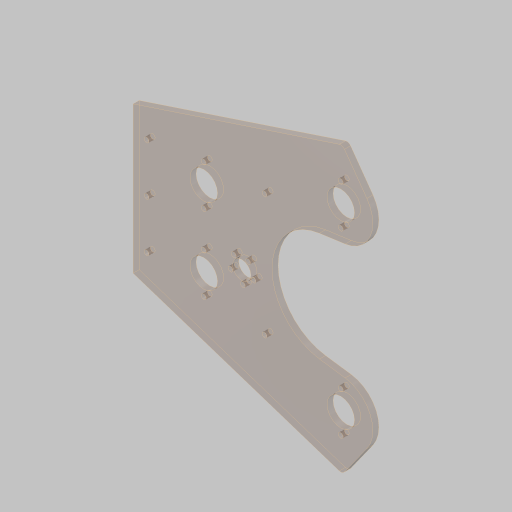
# Autodesk Inventor part: Part1
Saved by Autodesk Inventor 2023.5 (Build 275446000, 446)
## iProperties
Created: 2025-02-23
Part Number: Part1
Material: Polycarbonate, Smoke
Document SubType Name: Modeling
Designer: slick
Density: 1.2 g/cm^3
Appearance: Polycarbonate - Smoked
Author: slick
Autodesk Inventor part; units mm, degrees
ref_plane "YZ Plane" through (0, 0, 0) normal (1, 0, 0) x (0, 1, 0)
ref_plane "XZ Plane" through (0, 0, 0) normal (0, 1, 0) x (-1, 0, 0)
ref_plane "XY Plane" through (0, 0, 0) normal (0, 0, 1) x (1, 0, 0)
sketch "Sketch1" plane through (0, 0, 0) normal (0, 0, 1) x (1, 0, 0)
  circle A0 centre (0, 93.3256) radius 38.1 construction
  circle A1 centre (0, -93.3256) radius 38.1 construction
  line L0 (0, 93.3256) -> (0, -93.3256) construction
  circle A2 centre (-19.05, 0) radius 57.15 construction
  circle A3 centre (0, 93.3256) radius 14.2875
  circle A4 centre (0, -93.3256) radius 14.2875
  circle A5 centre (0, -93.3256) radius 33.3375 construction
  circle A6 centre (0, 93.3256) radius 33.3375 construction
  circle A7 centre (-142.4318, -39.6875) radius 14.3256 construction
  circle A8 centre (0, -93.3256) radius 23.876 construction
  line L1 (-142.4318, -39.6875) -> (0, -93.3256) construction
  circle A9 centre (-142.4318, 39.6875) radius 14.3256 construction
  circle A10 centre (0, 93.3256) radius 23.876 construction
  line L2 (0, 93.3256) -> (-142.4318, 39.6875) construction
  circle A11 centre (-142.4318, 39.6875) radius 39.6875 construction
  circle A12 centre (-142.4318, -39.6875) radius 39.6875 construction
  line L3 (-142.4318, 39.6875) -> (-142.4318, -39.6875) construction
  line L4 (-138.2343, 25.9906) -> (6.9958, 70.4975) construction
  line L5 (-9.8, 115.0976) -> (-148.3118, 52.7507) construction
  line L6 (-138.2343, -25.9906) -> (6.9958, -70.4975) construction
  line L7 (-13.7535, -112.8423) -> (-134.1797, -27.9775) construction
  circle A13 centre (-142.4318, 39.6875) radius 14.2875
  circle A14 centre (-142.4318, -39.6875) radius 14.2875
  circle A15 centre (-102.9059, -16.8672) radius 5.9531 construction
  circle A16 centre (-102.9059, -16.8672) radius 9.525
  circle A17 centre (-102.9059, -16.8672) radius 12.7 construction
  circle A18 centre (-102.9059, -16.8672) radius 12.7 construction
  circle A19 centre (-102.9059, -16.8672) radius 12.7 construction
  circle A20 centre (-102.9059, -16.8672) radius 12.7 construction
  circle A21 centre (-102.9059, -16.8672) radius 12.7 construction
  circle A22 centre (-14.2875, 0) radius 57.15 construction
  circle A23 centre (-102.9059, -16.8672) radius 19.05 construction
  line L8 (-215.9, 76.2) -> (-190.5, 76.2) construction
  line L9 (-190.5, 76.2) -> (-190.5, -76.2) construction
  line L10 (-190.5, -76.2) -> (-215.9, -76.2) construction
  line L11 (-215.9, -76.2) -> (-215.9, 76.2)
  line L12 (-142.4318, -39.6875) -> (-102.9059, -16.8672) construction
  line L13 (-79.1995, 63.5) -> (-79.1995, -63.5) construction
  line L14 (-22.1185, -56.6109) -> (4.5681, -60.3025)
  arc A24 (4.5681, 60.3025) -> (27.142, 112.6828) centre (0, 93.3256) ccw
  arc A25 (-22.1185, 56.6109) -> (-22.1185, -56.6109) centre (-14.2875, 0) ccw
  line L15 (4.5681, 60.3025) -> (-22.1185, 56.6109)
  arc A26 (27.142, -112.6828) -> (4.5681, -60.3025) centre (0, -93.3256) ccw
  arc A27 (3.8774, 145.3034) -> (-1.4945, 147.06) centre (0, 142.5381) ccw
  circle A28 centre (0, 93.3256) radius 44.45 construction
  line L16 (3.8774, 145.3034) -> (27.142, 112.6828)
  line L17 (-1.4945, 147.06) -> (-215.9, 76.2)
  arc A29 (-1.4945, -147.06) -> (3.8774, -145.3034) centre (0, -142.5381) ccw
  line L18 (-215.9, -76.2) -> (-1.4945, -147.06)
  line L19 (27.142, -112.6828) -> (3.8774, -145.3034)
  circle A30 centre (0, -93.3256) radius 44.45 construction
  line L20 (0, 114.3441) -> (0, 72.3071) construction
  line L21 (-142.4318, 60.706) -> (-142.4318, 18.669) construction
  line L22 (-142.4318, -18.669) -> (-142.4318, -60.706) construction
  line L23 (0, -72.3071) -> (0, -114.3441) construction
  line L24 (-201.797, 50.8) -> (-201.797, -50.8) construction
  point P0 (0, 0)
  point P1 (0, 0)
  point P2 (-111.2471, -7.2904)
  point P3 (-114.5915, -21.8408)
  point P4 (-101.7868, -29.5178)
  point P5 (-90.5286, -19.7121)
  point P6 (-96.3754, -5.9749)
  point P7 (-190.5, 0)
  point P8 (-201.797, 0)
  point P9 (-201.797, 0)
  dimension "d15" = 25.4
  dimension "d0" = 76.2
  dimension "d1" = 76.2
  dimension "d2" = 114.3
  dimension "d4" = 186.6511
  dimension "d5" = 28.575
  dimension "d6" = 19.05
  dimension "d7" = 28.6512
  dimension "d8" = 47.752
  dimension "d9" = 79.375
  dimension "d10" = 142.4318
  dimension "d11" = 152.1968
  dimension "d12" = 28.575
  dimension "d13" = 11.9062
  dimension "d14" = 19.05
  dimension "d18" = 360
  dimension "d20" = 4.7625
  dimension "d21" = 38.1
  dimension "d22" = 25.4
  dimension "d23" = 152.4
  dimension "d24" = 215.9
  dimension "d25" = 60
  dimension "d26" = 127
  dimension "d29" = 9.525
  dimension "d30" = 6.35
  dimension "d32" = 42.037
  dimension "d33" = 42.037
  dimension "d34" = 42.037
  dimension "d35" = 42.037
  dimension "d36" = 19.05
  dimension "d44" = 101.6
  constraints: 50 end point, 26 centre point, 24 point on circle, 24 tangent, 16 coincident, 9 equal radius, 8 vertical, 7 midpoint, 3 horizontal alignment, 2 parallel, 2 point on line, 2 vertical alignment, 1 equal length, 1 horizontal, 1 perpendicular, 31 other
  measures "d0" diameter of A0
  measures "d1" diameter of A1
  measures "d2" diameter of A2
  measures "d4" distance of L0.end L0.start
  measures "d5" diameter of A3
  measures "d6" radial gap between concentric circles of A4 A5
  measures "d7" diameter of A7
  measures "d8" diameter of A8
  measures "d9" diameter of A11
  measures "d10" distance from line of L0.start L3
  measures "d11" distance of L2.end L2.start
  measures "d12" diameter of A13
  measures "d13" diameter of A15
  measures "d14" diameter of A16
  measures "d20" distance of A2.centre A22.centre
  measures "d21" diameter of A23
  measures "d22" distance of L9.end L10.end
  measures "d23" distance of L10.end L8.start
  measures "d24" distance from line of A3.centre L11
  measures "d25" angle of L12 L3
  measures "d26" distance of L13.start L13.end
  measures "d29" diameter of A27
  measures "d30" radial gap between concentric circles of A0 A28
  measures "d32" distance of L20.start L20.end
  measures "d33" distance of L21.start L21.end
  measures "d34" distance of L22.start L22.end
  measures "d35" distance of L23.start L23.end
  measures "d36" distance of point (0, 0) A2.centre
  measures "d44" distance of L24.start L24.end
extrude "Extrusion1" add sketch "Sketch1" along normal blind 6.35
hole "Hole1" at (-111.2471, -7.2904, 0) at (-114.5915, -21.8408, 0) at (-101.7868, -29.5178, 0) at (-90.5286, -19.7121, 0) at (-96.3754, -5.9749, 0) at (-79.1995, 63.5, 0) at (-79.1995, -63.5, 0) at (0, 114.3441, 0) at (0, 72.3071, 0) at (-142.4318, 60.706, 0) at (-142.4318, 18.669, 0) at (-142.4318, -18.669, 0) at (-142.4318, -60.706, 0) at (0, -72.3071, 0) at (0, -114.3441, 0) at (-201.797, 50.8, 0) at (-201.797, 0, 0) at (-201.797, -50.8, 0) direction (0, 0, 1) diameter 5.1054 end through all clearance for "Flat Head Machine Screw (82)" size "#10" standard "Ansi Unified Screw Threads"
body "Solid1"
